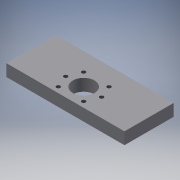
# Autodesk Inventor part: CHAPA_APOIO_CASTANHA_EIXO_Z
Saved by Autodesk Inventor 2018 (Build 220112000, 112)
## iProperties
Created: 2018-10-11
Part Number: CHAPA_APOIO_CASTANHA_EIXO_Z
Material: Genérico
Document SubType Name: Modeling
Designer: Usuario
Density: 1 g/cm^3
Appearance: Padrão
Author: Usuario
Autodesk Inventor part; units mm, degrees
ref_plane "YZ Plane" through (0, 0, 0) normal (1, 0, 0) x (0, 1, 0)
ref_plane "XZ Plane" through (0, 0, 0) normal (0, 1, 0) x (-1, 0, 0)
ref_plane "XY Plane" through (0, 0, 0) normal (0, 0, 1) x (1, 0, 0)
sketch "Esboço1" plane through (0, 0, 0) normal (0, 0, 1) x (1, 0, 0)
  line L0 (0, 12.7) -> (125, 12.7)
  line L1 (125, 12.7) -> (125, -39.3)
  line L2 (125, -39.3) -> (0, -39.3)
  line L3 (0, -39.3) -> (0, 12.7)
  circle A0 centre (62.5, -20) radius 11.5
  dimension "d0" = 52
  dimension "d1" = 23
  dimension "d2" = 125
  constraints: 8 end point, 2 parallel, 1 centre point, 1 horizontal, 1 perpendicular
  measures "d0" distance of L0.end L1.end
  measures "d1" diameter of A0
  measures "d2" distance of L1.end L2.end
extrude "Extrusão1" add sketch "Esboço1" along normal blind 12.7
sketch "Esboço3" plane through (0, 0, 12.7) normal (0, 0, 1) x (1, 0, 0)
  circle A0 centre (75.935, -33.435) radius 2.75 construction
  circle A1 centre (49.065, -33.435) radius 2.75 construction
  circle A2 centre (81.5, -20) radius 2.75 construction
  circle A3 centre (43.5, -20) radius 2.75 construction
  circle A4 centre (49.065, -6.565) radius 2.75 construction
  circle A5 centre (75.935, -6.565) radius 2.75 construction
  point P0 (0, 0)
  constraints: 6 centre point
hole "Furo2" at (75.935, -33.435, 12.7) at (49.065, -33.435, 12.7) at (81.5, -20, 12.7) at (43.5, -20, 12.7) at (49.065, -6.565, 12.7) at (75.935, -6.565, 12.7) direction (0, 0, -1) diameter 4.134 end through all thread size "M5x0.8" class "6H" standard "ANSI Metric M Profile"
sketch "Esboço5" plane through (0, 0, 12.7) normal (0, 0, 1) x (1, 0, 0)
  circle A0 centre (6.5, 6.35) radius 2.067
  circle A1 centre (34.5, 6.35) radius 2.067
  circle A2 centre (62.5, 6.35) radius 2.067
  circle A3 centre (90.5, 6.35) radius 2.067
  circle A4 centre (118.5, 6.35) radius 2.067
  point P0 (0, 0)
  constraints: 5 centre point
hole "Furo3" at (6.5, 6.35, 12.7) at (34.5, 6.35, 12.7) at (62.5, 6.35, 12.7) at (90.5, 6.35, 12.7) at (118.5, 6.35, 12.7) direction (0, 0, -1) diameter 5.5 end through all counterbore diameter 8 counterbore depth 6
